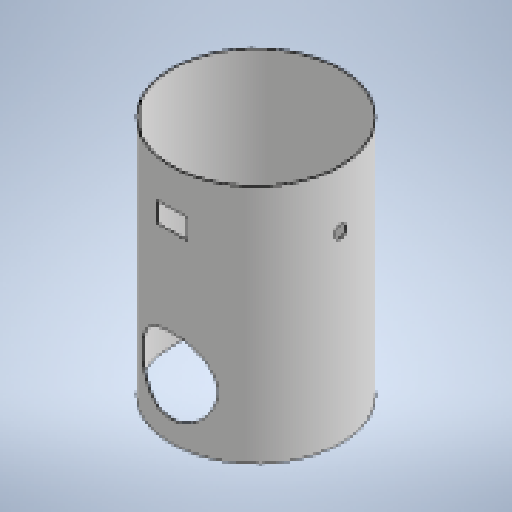
# Autodesk Inventor part: PRS 0101 main shell D1200
Saved by Autodesk Inventor 2026.2 (Build 302298010, 298A)
## iProperties
Created: 2025-02-11
Part Number: PRS 0101 main shell D1200
Material: Steel
Document SubType Name: Sheet Metal
Designer: pokla
Mass: 287778 g
Surface Area: 123017 cm^2
Volume: 36659.6 cm^3
Density: 7.85 g/cm^3
Flat Pattern Width: 170 cm
Flat Pattern Length: 172.811 cm
Flat Pattern Area: 29377.9 cm^2
Sheet Metal Rule: Default_mm
Sheet Metal Width: 1700,000 mm
Sheet Metal Length: 1728,114 mm
Sheet Metal Area: 2937793,546 mm^2
Appearance: Default
AA_MAIN_filter_diam: 1200,000 mm
Legs_Tube_lenght: 413,666 mm
Legs_Tube_cut_angle: 25,90 grad
Legs_Tube_dim: 80,000 mm
Legs_Upper_plate_lenght: 122,110 mm
Legs_Inner_diam: 880,000 mm
AA_MAIN_Filter_Clearance: 300,000 mm
ChargingHatch_width: 208,000 mm
ChargingHatch_hight: 122,000 mm
AccsessHatch_tube_diameter: 530,000 mm
Author: pokla
Autodesk Inventor part; units mm, degrees
note: some values were not read from the file. Left out: dimensions or parameters whose unit could not be read.
sketch "Sketch13" plane through (0, 0, 0) normal (0, 0, 1) x (1, 0, 0)
  circle A0 centre (0, 0) radius 600 construction
  line L0 (0, 0) -> (0, -600)
  line L1 (0, 0) -> (-519.6152, -300)
  line L2 (0, 0) -> (600, 0)
  line L3 (0, 0) -> (0, -600)
  line L4 (0, 0) -> (0, -600)
  line L5 (0, 0) -> (534.6039, 272.3943)
  line L6 (0, 0) -> (0, 600)
  dimension "d53" = 1200
  dimension "d55" = 0
  dimension "d98" = 180
  dimension "d99" = 240
  dimension "d100" = 63
  dimension "d101" = 90
  constraints: 14 end point, 1 coincident, 1 point on line, 1 vertical, 9 other
  measures "d55" distance between parallel lines of L0 L4
  measures "d98" angle of L3 L6
  measures "d100" angle of L6 L5
  measures "d101" angle of L2 L6
ref_plane "WeldJoint" through (0, 0, -10) normal (0.5, -0.866, 0) x (0, 0, 1)
ref_plane "Inlet_Clock_Angle_plane" through (0, 0, -10) normal (0, 1, 0) x (0, 0, 1)
ref_plane "Charging" through (0, 0, -10) normal (1, 0, 0) x (0, 0, 1)
ref_plane "Accsess" through (0, 0, -10) normal (1, 0, 0) x (0, 0, 1)
sketch "Sketch14" plane through (0, 0, -10) normal (0.5, -0.866, 0) x (0, 0, 1)
  line L0 (1710, 594) -> (10, 594)
  line L1 (10, 594) -> (10, 600)
  line L2 (10, 600) -> (1710, 600)
  line L3 (1710, 600) -> (1710, 594)
  line L4 (10, 0) -> (1710, 0)
  line L5 (10, 600) -> (-20, 600) construction
  line L6 (10, 594) -> (-20, 594) construction
  arc A0 (-20, 594) -> (-109.2789, 539.0476) centre (-20, 494) ccw construction
  arc A1 (-109.2789, 539.0476) -> (-234, 15) centre (929.3202, 15) ccw construction
  line L7 (-234, 15) -> (-234, 0) construction
  line L8 (10, 0) -> (-234, 0) construction
  arc A2 (-20, 600) -> (-114.6356, 541.7504) centre (-20, 494) ccw construction
  arc A3 (-114.6356, 541.7504) -> (-240, 15) centre (929.3202, 15) ccw construction
  line L9 (-240, 15) -> (-240, 0) construction
  line L10 (-234, 0) -> (-240, 0) construction
  line L11 (1710, 594) -> (1740, 594)
  line L12 (1710, 600) -> (1740, 600)
  line L13 (1710, 0) -> (1954, 0) construction
  line L14 (1960, 0) -> (1960, 15) construction
  arc A4 (1960, 15) -> (1834.6356, 541.7504) centre (790.6798, 15) ccw construction
  arc A5 (1834.6356, 541.7504) -> (1740, 600) centre (1740, 494) ccw construction
  line L15 (1954, 0) -> (1954, 15) construction
  line L16 (1954, 0) -> (1960, 0) construction
  arc A6 (1954, 15) -> (1829.2789, 539.0476) centre (790.6798, 15) ccw construction
  arc A7 (1829.2789, 539.0476) -> (1740, 594) centre (1740, 494) ccw construction
  line L17 (-160.8038, 520) -> (-540, 520)
  line L18 (-540, 520) -> (-540, 440)
  line L19 (-540, 440) -> (-160.8038, 440)
  line L20 (-160.8038, 440) -> (-160.8038, 520)
  line L21 (1960, 15) -> (1990, 15) construction
  line L22 (1990, 15) -> (1990, 0) construction
  line L23 (1990, 0) -> (1960, 0) construction
  line L24 (-540, 600) -> (-540, 520)
  line L25 (-540, 600) -> (-534, 600)
  line L26 (-534, 600) -> (-534, 520)
  line L27 (-120.3984, 533.7757) -> (-168.7178, 421.6324)
  line L28 (-160.8038, 520) -> (-126.334, 520)
  line L29 (-109.2789, 539.0476) -> (-114.6356, 541.7504)
  line L30 (-120.3984, 533.7757) -> (-116.5468, 542.7148) construction
  line L31 (-116.5468, 542.7148) -> (-114.6356, 541.7504) construction
  line L32 (-540, 600) -> (-540, 600)
  line L33 (-540, 600) -> (-540, 440)
  line L34 (-540, 440) -> (-540, 440)
  line L35 (1355, 600) -> (1265, 600)
  line L36 (1265, 600) -> (1265, 700)
  line L37 (1265, 700) -> (1355, 700)
  line L38 (1355, 700) -> (1355, 600)
  point P0 (10, 597)
  point P1 (-144.5581, 477.7041)
  point P2 (1310, 700)
  dimension "d59" = 1700
  dimension "d60" = 6
  dimension "d61" = 1200
  dimension "d82" = 100
  dimension "d83" = 30
  dimension "d86" = 80
  dimension "d87" = 30
  dimension "d91" = 15
  dimension "d92" = 20
  dimension "d93" = 250
  dimension "d94" = 30
  dimension "d103" = 413.666
  dimension "d104" = 23.31
  dimension "d105" = 122.1101
  dimension "d107" = 9.7336
  dimension "d108" = 880
  dimension "d109" = 0
  dimension "d110" = 2530
  dimension "d111" = 300
  dimension "d112" = 100
  dimension "d113" = 90
  dimension "d114" = 1850
  dimension "d115" = 1300
  dimension "d116" = 80
  constraints: 78 end point, 18 point on circle, 14 horizontal, 13 tangent, 10 perpendicular, 8 centre point, 7 point on line, 6 equal length, 6 parallel, 4 concentric, 3 midpoint, 2 collinear, 2 equal radius, 2 vertical, 1 vertical alignment
  measures "d59" distance of L1.end L2.end
  measures "d60" distance of L0.end L1.end
  measures "d61" diameter of L2 L4
  measures "d82" radius of A0
  measures "d83" distance of L0.end L6.end
  measures "d86" distance of L17.end L18.end
  measures "d87" distance of L14.end L21.end
  measures "d91" distance of L28.end L27.start
  measures "d92" distance of L19.end L27.end
  measures "d93" distance of L9.end L4.start
  measures "d94" diameter of L9.start L4
  measures "d103" distance from line of L18 L28.end
  measures "d104" angle of L20 L27
  measures "d105" distance of L27.end L27.start
  measures "d107" distance of L27.start L30.end
  measures "d108" diameter of L19 L4
  measures "d109" distance of L24.start L32.end
  measures "d110" distance between parallel lines of L33 L22
  measures "d111" distance between parallel lines of L9 L33
  measures "d112" distance of L37.end L35.start
  measures "d113" distance of L36.end L37.end
  measures "d114" distance from line of L33 point (1310, 700)
  measures "d115" distance from line of L1 point (1310, 700)
  measures "d116" distance between parallel lines of L17 L2
revolve "Revolution2" add sketch "Sketch14" angle 359.9 about axis through (0, 0, 0) along (0, 0, 1) contours L0 L1 L2 L3
sketch "Sketch AnglePlane_InletPipe" plane through (0, 0, -10) normal (0, 1, 0) x (0, 0, 1)
  line L0 (10, -600) -> (10, 600) projected
  line L1 (10, 0) -> (1310, 0)
  line L2 (1310, 0) -> (1310, 600)
  line L3 (1310, 600) -> (10, 600)
  line L4 (10, 600) -> (10, 0)
  point P0 (10, -519.6152)
  point P1 (10, -520.138)
  dimension "d63" = 1200
  dimension "d64" = 90
  dimension "frd_hght" = 1300
  constraints: 8 end point, 1 collinear, 1 horizontal, 1 parallel
  measures "d63" diameter of L3 L1
  measures "d64" angle of L2 L3
  measures "frd_hght" distance of L2.end L3.end
ref_plane "InletPipe_AnglePlane" through (0, 0, 1300) normal (1, 0, 0) x (0, 1, 0)
sketch "Sketch16" plane through (0, 0, 1300) normal (1, 0, 0) x (0, 1, 0)
  circle A0 centre (0, 0) radius 45.5
  point P0 (0, -1300)
  point P1 (0, 0)
  point P2 (0, 0)
  point P3 (0, 0)
  dimension "d66" = 91
  constraints: 1 centre point, 1 coincident
  measures "d66" diameter of A0
extrude "Extrusion7" cut sketch "Sketch16" along normal through all
ref_plane "Work Plane16" through (0, 0, 0) normal (0, -1, 0) x (1, 0, 0)
sketch "Sketch17" plane through (0, 0, 0) normal (0, -1, 0) x (1, 0, 0)
  circle A0 centre (0, 416) radius 266
  line L0 (0, 150) -> (-495.5727, 150)
  point P0 (0, 0)
  dimension "d69" = 532
  dimension "d71" = 150
  constraints: 2 end point, 2 horizontal, 2 vertical alignment, 2 other
  measures "d71" distance from line of point (0, 0) L0
extrude "Extrusion8" cut sketch "Sketch17" along normal through all
sketch "ChargingAngleSketch19" plane through (0, 0, -10) normal (1, 0, 0) x (0, 0, 1)
  line L0 (10, 0) -> (963.5898, 0)
  line L1 (963.5898, 0) -> (1310, 600)
  line L2 (1310, 600) -> (10, 600)
  line L3 (10, 600) -> (10, 0)
  dimension "d74" = 1300
  dimension "d76" = 1200
  dimension "d77" = 60
  constraints: 8 end point, 1 horizontal, 1 parallel, 1 perpendicular
  measures "d74" distance of L1.end L2.end
  measures "d76" diameter of L2 L0
  measures "d77" angle of L2 L1
ref_plane "Work Plane18" through (0, 0, 953.5898) normal (0, -0.866, 0.5) x (1, 0, 0)
sketch "Sketch20" plane through (0, 0, 953.5898) normal (0, -0.866, 0.5) x (1, 0, 0)
  line L0 (-104, 0) -> (104, 0)
  line L1 (104, 0) -> (104, 122)
  line L2 (104, 122) -> (-104, 122)
  line L3 (-104, 122) -> (-104, 0)
  point P0 (0, -825.833)
  point P1 (0, 0)
  point P2 (0, 0)
  point P3 (0, 0)
  point P4 (0, 0)
  dimension "d78" = 208
  dimension "d79" = 122
  constraints: 8 end point, 2 parallel, 1 coincident, 1 horizontal, 1 midpoint, 1 perpendicular
  measures "d78" distance of L2.end L1.end
  measures "d79" distance of L1.end L0.end
extrude "Charging hole" cut sketch "Sketch20" along normal through all
sketch "Sketch1" plane through (0, -1700, 0) normal (0, 0, 1) x (1, 0, 0)
  line L0 (520.8574, 1294.7565) -> (520.8574, 1435.6299) projected
  line L1 (728.7425, 1435.6299) -> (728.7425, 1294.7565) projected
  line L2 (532.8574, 1424.7204) -> (532.8574, 1307.9421)
  line L3 (716.7425, 1307.9421) -> (716.7425, 1424.7204)
  line L4 (624.7999, 682) -> (624.7999, 150) construction
  line L5 (350.7548, 416) -> (898.8451, 416) construction
  line L6 (1728.1139, 1564.2642) -> (1182.3519, -339.0339)
  line L7 (1182.3519, -339.0339) -> (0, 0)
  line L8 (0, 0) -> (545.762, 1903.2982)
  line L9 (545.762, 1903.2982) -> (1728.1139, 1564.2642)
  line L10 (1728.1139, 1564.2642) -> (0, 0) construction
  line L11 (1182.3519, -339.0339) -> (545.762, 1903.2982) construction
  line L12 (0, 0) -> (1279.5683, 0)
  line L13 (0, 1700) -> (0, 0) projected
  line L14 (0, 0) -> (3747.7583, 0) projected
  line L15 (0, 1700) -> (3747.7583, 1700) projected
  line L16 (3747.7583, 1700) -> (3747.7583, 0) projected
  ellipse E0 centre (624.7999, 416) end of major axis (624.7999, 150) minor radius 279
  line L17 (509.8574, 1445.5785) -> (509.8574, 1282.5939)
  line L18 (739.7425, 1282.5939) -> (739.7425, 1445.5785)
  point P0 (864.0569, 782.1321)
  point P1 (1516.7112, 1300)
  point P2 (1607.2885, 1300)
  point P3 (1595.2885, 1300)
  point P4 (1528.7112, 1300)
  point P5 (1254.7469, 1700)
  point P6 (487.4672, 1700)
  point P7 (729.8034, 1432.112)
  point P8 (519.7965, 1432.112)
  point P9 (520.8574, 1432.2183)
  point P10 (728.7425, 1432.2183)
  point P11 (1618.2885, 1300)
  point P12 (1505.7112, 1300)
  dimension "d0" = 12
  dimension "d10" = 12
  dimension "d13" = 279
  dimension "d15" = 11
  dimension "d16" = 11
  dimension "d17" = 11
  dimension "d3" = 532
  dimension "d4" = 548.0902
  dimension "d6" = 1980
  dimension "d8" = 1230
  dimension "d9" = 16
  dimension "d14" = 12
  constraints: 26 end point, 12 horizontal alignment, 8 parallel, 4 midpoint, 2 horizontal, 2 vertical, 1 coincident, 1 perpendicular, 1 point on line, 24 other
  measures "d3" distance of L4.start L4.end
  measures "d4" distance of L5.start L5.end
  measures "d6" distance of L6.start L6.end
  measures "d8" distance of L7.end L6.end
  measures "d9" angle of L13 L8
equation "\"BendRadius\" = Thickness"
equation "\"BendReliefWidth\" = Thickness"
equation "\"BendReliefDepth\" = 0.5 * Thickness"
equation "\"CornerReliefSize\" = 4 * Thickness"
equation "\"MinimumRemnant\" = 2 * Thickness"
equation "\"TransitionRadius\" = BendRadius"
equation "\"JacobiRadiusSize\" = BendRadius"
equation "\"GapSize\" = Thickness"
equation "\"InletPipe_horisont_angle\" = 0"
equation "\"ChargingHatch_width\" = 208"
equation "\"ChargingHatch_hight\" = 122"
equation "\"AccsessHatch_ClockAngle\" = 0"
equation "\"ChargingHatch_ClockAgnle\" = 180deg"
equation "\"InletPipe_Clock_angle\" = 90deg"
equation "\"OutletPipe_ClockAngle\" = 63deg"
equation "\"WeldJoint_ClockAgnle\" = 240deg"
equation "\"Legs_Tube_lenght\" = 413.666"
equation "\"Legs_Upper_plate_lenght\" = 122.11007"
equation "\"Thickness\" = 6"
body "Solid2"
